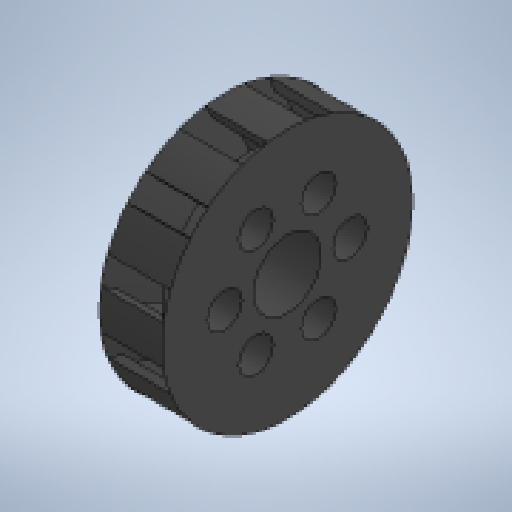
# Autodesk Inventor part: Idler - Hub
Saved by Autodesk Inventor 2023.2 (Build 272271000, 271)
## iProperties
Created: 2023-11-16
Part Number: Idler - Hub
Material: Nylon 6/6
Document SubType Name: Modeling
Designer: Nathan Cai
Density: 1.13 g/cm^3
Appearance: Rubber - Black
Author: Nathan Cai
Autodesk Inventor part; units mm, degrees
ref_plane "YZ Plane" through (0, 0, 0) normal (1, 0, 0) x (0, 1, 0)
ref_plane "XZ Plane" through (0, 0, 0) normal (0, 1, 0) x (-1, 0, 0)
ref_plane "XY Plane" through (0, 0, 0) normal (0, 0, 1) x (1, 0, 0)
sketch "Sketch1" plane through (0, 0, 0) normal (0, 0, 1) x (1, 0, 0)
  line L0 (-3.175, -12.7) -> (3.175, -12.7)
  line L1 (3.175, -12.7) -> (3.175, 12.7)
  line L2 (3.175, 12.7) -> (-3.175, 12.7)
  line L3 (-3.175, 12.7) -> (-3.175, -12.7)
  line L4 (-3.175, -12.7) -> (3.175, 12.7) construction
  line L5 (3.175, -12.7) -> (-3.175, 12.7) construction
  line L6 (-3.175, 0) -> (3.175, 0) construction
  line L7 (-3.175, -3.429) -> (3.175, -3.429)
  line L8 (3.175, -3.429) -> (3.175, 3.429)
  line L9 (3.175, 3.429) -> (-3.175, 3.429)
  line L10 (-3.175, 3.429) -> (-3.175, -3.429)
  line L11 (-3.175, -3.429) -> (3.175, 3.429) construction
  line L12 (3.175, -3.429) -> (-3.175, 3.429) construction
  line L13 (-1.5875, 9.525) -> (1.5875, 9.525)
  line L14 (1.5875, 9.525) -> (1.5875, 15.875)
  line L15 (1.5875, 15.875) -> (-1.5875, 15.875)
  line L16 (-1.5875, 15.875) -> (-1.5875, 9.525)
  line L17 (-1.5875, 9.525) -> (1.5875, 15.875) construction
  line L18 (1.5875, 9.525) -> (-1.5875, 15.875) construction
  point P0 (0, 0)
  point P1 (0, 12.7)
  point P2 (-1.5875, 12.7)
  point P3 (1.5875, 12.7)
  dimension "d0" = 6.35
  dimension "d1" = 25.4
  dimension "d2" = 6.35
  dimension "d3" = 6.858
  dimension "d4" = 3.175
  dimension "d5" = 6.35
  constraints: 38 end point, 9 midpoint, 6 parallel, 3 horizontal, 3 perpendicular
  measures "d0" distance of L2.end L1.end
  measures "d1" distance of L1.end L0.end
  measures "d2" distance of L9.end L8.end
  measures "d3" distance of L8.end L7.end
  measures "d4" distance of L15.end L14.end
  measures "d5" distance of L14.end L13.end
revolve "Revolution1" add sketch "Sketch1" angle 360 about axis through (-3.175, 0, 0) along (1, 0, 0) contours L3 L2 L16 L13 L14 L1 L9
chamfer "Chamfer1" distance 1.5875 angle 45 4 edges at (-1.5875, -12.7, 0) (1.5875, -12.7, 0) (-1.5875, -9.525, 0) (1.5875, -9.525, 0)
sketch "Sketch2" plane through (3.175, 0, 0) normal (1, 0, 0) x (0, 0, -1)
  circle A0 centre (0, 0) radius 9.525
  arc A1 (-11.7597, 1.8625) -> (-11.7597, -1.8625) centre (0, 0) ccw
  circle A2 centre (0, 0) radius 12.7 projected
  line L0 (-12.7, 0) -> (0, 0) construction
  line L1 (-9.5064, -0.5953) -> (-11.8914, -0.5953)
  line L2 (-11.8914, -0.5953) -> (-11.8914, 0.5953) construction
  line L3 (-11.8914, 0.5953) -> (-9.5064, 0.5953)
  line L4 (-9.5064, 0.5953) -> (-9.5064, -0.5953) construction
  line L5 (-9.5064, -0.5953) -> (-11.8914, 0.5953) construction
  line L6 (-11.8914, -0.5953) -> (-9.5064, 0.5953) construction
  line L7 (0, 0) -> (-12.5436, 1.9867) construction
  line L8 (-11.7597, 1.8625) -> (-12.5436, 1.9867)
  line L9 (-11.7597, -1.8625) -> (-12.5436, -1.9867)
  arc A3 (-11.1154, -4.2668) -> (-9.2529, -7.4928) centre (0, 0) ccw
  line L10 (-7.9351, -5.2687) -> (-10.0006, -6.4612)
  line L11 (-10.0006, -6.4612) -> (-10.5959, -5.4301) construction
  line L12 (-10.5959, -5.4301) -> (-8.5304, -4.2376)
  line L13 (-8.5304, -4.2376) -> (-7.9351, -5.2687) construction
  line L14 (-7.9351, -5.2687) -> (-10.5959, -5.4301) construction
  line L15 (-10.0006, -6.4612) -> (-8.5304, -4.2376) construction
  line L16 (-11.1154, -4.2668) -> (-11.8565, -4.5513)
  line L17 (-9.2529, -7.4928) -> (-9.8698, -7.9924)
  arc A4 (-7.4928, -9.2529) -> (-4.2668, -11.1154) centre (0, 0) ccw
  line L18 (-4.2376, -8.5304) -> (-5.4301, -10.5959)
  line L19 (-5.4301, -10.5959) -> (-6.4612, -10.0006) construction
  line L20 (-6.4612, -10.0006) -> (-5.2687, -7.9351)
  line L21 (-5.2687, -7.9351) -> (-4.2376, -8.5304) construction
  line L22 (-4.2376, -8.5304) -> (-6.4612, -10.0006) construction
  line L23 (-5.4301, -10.5959) -> (-5.2687, -7.9351) construction
  line L24 (-7.4928, -9.2529) -> (-7.9924, -9.8698)
  line L25 (-4.2668, -11.1154) -> (-4.5513, -11.8565)
  arc A5 (-1.8625, -11.7597) -> (1.8625, -11.7597) centre (0, 0) ccw
  line L26 (0.5953, -9.5064) -> (0.5953, -11.8914)
  line L27 (0.5953, -11.8914) -> (-0.5953, -11.8914) construction
  line L28 (-0.5953, -11.8914) -> (-0.5953, -9.5064)
  line L29 (-0.5953, -9.5064) -> (0.5953, -9.5064) construction
  line L30 (0.5953, -9.5064) -> (-0.5953, -11.8914) construction
  line L31 (0.5953, -11.8914) -> (-0.5953, -9.5064) construction
  line L32 (-1.8625, -11.7597) -> (-1.9867, -12.5436)
  line L33 (1.8625, -11.7597) -> (1.9867, -12.5436)
  arc A6 (4.2668, -11.1154) -> (7.4928, -9.2529) centre (0, 0) ccw
  line L34 (5.2687, -7.9351) -> (6.4612, -10.0006)
  line L35 (6.4612, -10.0006) -> (5.4301, -10.5959) construction
  line L36 (5.4301, -10.5959) -> (4.2376, -8.5304)
  line L37 (4.2376, -8.5304) -> (5.2687, -7.9351) construction
  line L38 (5.2687, -7.9351) -> (5.4301, -10.5959) construction
  line L39 (6.4612, -10.0006) -> (4.2376, -8.5304) construction
  line L40 (4.2668, -11.1154) -> (4.5513, -11.8565)
  line L41 (7.4928, -9.2529) -> (7.9924, -9.8698)
  arc A7 (9.2529, -7.4928) -> (11.1154, -4.2668) centre (0, 0) ccw
  line L42 (8.5304, -4.2376) -> (10.5959, -5.4301)
  line L43 (10.5959, -5.4301) -> (10.0006, -6.4612) construction
  line L44 (10.0006, -6.4612) -> (7.9351, -5.2687)
  line L45 (7.9351, -5.2687) -> (8.5304, -4.2376) construction
  line L46 (8.5304, -4.2376) -> (10.0006, -6.4612) construction
  line L47 (10.5959, -5.4301) -> (7.9351, -5.2687) construction
  line L48 (9.2529, -7.4928) -> (9.8698, -7.9924)
  line L49 (11.1154, -4.2668) -> (11.8565, -4.5513)
  arc A8 (11.7597, -1.8625) -> (11.7597, 1.8625) centre (0, 0) ccw
  line L50 (9.5064, 0.5953) -> (11.8914, 0.5953)
  line L51 (11.8914, 0.5953) -> (11.8914, -0.5953) construction
  line L52 (11.8914, -0.5953) -> (9.5064, -0.5953)
  line L53 (9.5064, -0.5953) -> (9.5064, 0.5953) construction
  line L54 (9.5064, 0.5953) -> (11.8914, -0.5953) construction
  line L55 (11.8914, 0.5953) -> (9.5064, -0.5953) construction
  line L56 (11.7597, -1.8625) -> (12.5436, -1.9867)
  line L57 (11.7597, 1.8625) -> (12.5436, 1.9867)
  arc A9 (11.1154, 4.2668) -> (9.2529, 7.4928) centre (0, 0) ccw
  line L58 (7.9351, 5.2687) -> (10.0006, 6.4612)
  line L59 (10.0006, 6.4612) -> (10.5959, 5.4301) construction
  line L60 (10.5959, 5.4301) -> (8.5304, 4.2376)
  line L61 (8.5304, 4.2376) -> (7.9351, 5.2687) construction
  line L62 (7.9351, 5.2687) -> (10.5959, 5.4301) construction
  line L63 (10.0006, 6.4612) -> (8.5304, 4.2376) construction
  line L64 (11.1154, 4.2668) -> (11.8565, 4.5513)
  line L65 (9.2529, 7.4928) -> (9.8698, 7.9924)
  arc A10 (7.4928, 9.2529) -> (4.2668, 11.1154) centre (0, 0) ccw
  line L66 (4.2376, 8.5304) -> (5.4301, 10.5959)
  line L67 (5.4301, 10.5959) -> (6.4612, 10.0006) construction
  line L68 (6.4612, 10.0006) -> (5.2687, 7.9351)
  line L69 (5.2687, 7.9351) -> (4.2376, 8.5304) construction
  line L70 (4.2376, 8.5304) -> (6.4612, 10.0006) construction
  line L71 (5.4301, 10.5959) -> (5.2687, 7.9351) construction
  line L72 (7.4928, 9.2529) -> (7.9924, 9.8698)
  line L73 (4.2668, 11.1154) -> (4.5513, 11.8565)
  arc A11 (1.8625, 11.7597) -> (-1.8625, 11.7597) centre (0, 0) ccw
  line L74 (-0.5953, 9.5064) -> (-0.5953, 11.8914)
  line L75 (-0.5953, 11.8914) -> (0.5953, 11.8914) construction
  line L76 (0.5953, 11.8914) -> (0.5953, 9.5064)
  line L77 (0.5953, 9.5064) -> (-0.5953, 9.5064) construction
  line L78 (-0.5953, 9.5064) -> (0.5953, 11.8914) construction
  line L79 (-0.5953, 11.8914) -> (0.5953, 9.5064) construction
  line L80 (1.8625, 11.7597) -> (1.9867, 12.5436)
  line L81 (-1.8625, 11.7597) -> (-1.9867, 12.5436)
  arc A12 (-4.2668, 11.1154) -> (-7.4928, 9.2529) centre (0, 0) ccw
  line L82 (-5.2687, 7.9351) -> (-6.4612, 10.0006)
  line L83 (-6.4612, 10.0006) -> (-5.4301, 10.5959) construction
  line L84 (-5.4301, 10.5959) -> (-4.2376, 8.5304)
  line L85 (-4.2376, 8.5304) -> (-5.2687, 7.9351) construction
  line L86 (-5.2687, 7.9351) -> (-5.4301, 10.5959) construction
  line L87 (-6.4612, 10.0006) -> (-4.2376, 8.5304) construction
  line L88 (-4.2668, 11.1154) -> (-4.5513, 11.8565)
  line L89 (-7.4928, 9.2529) -> (-7.9924, 9.8698)
  arc A13 (-9.2529, 7.4928) -> (-11.1154, 4.2668) centre (0, 0) ccw
  line L90 (-8.5304, 4.2376) -> (-10.5959, 5.4301)
  line L91 (-10.5959, 5.4301) -> (-10.0006, 6.4612) construction
  line L92 (-10.0006, 6.4612) -> (-7.9351, 5.2687)
  line L93 (-7.9351, 5.2687) -> (-8.5304, 4.2376) construction
  line L94 (-8.5304, 4.2376) -> (-10.0006, 6.4612) construction
  line L95 (-10.5959, 5.4301) -> (-7.9351, 5.2687) construction
  line L96 (-9.2529, 7.4928) -> (-9.8698, 7.9924)
  line L97 (-11.1154, 4.2668) -> (-11.8565, 4.5513)
  circle A14 centre (0, 0) radius 3.429
  point P0 (-10.6989, 0)
  point P1 (-10.9985, -6.35)
  point P2 (-9.2655, -5.3494)
  point P3 (-6.35, -10.9985)
  point P4 (-5.3494, -9.2655)
  point P5 (0, -12.7)
  point P6 (0, -10.6989)
  point P7 (6.35, -10.9985)
  point P8 (5.3494, -9.2655)
  point P9 (10.9985, -6.35)
  point P10 (9.2655, -5.3494)
  point P11 (12.7, 0)
  point P12 (10.6989, 0)
  point P13 (10.9985, 6.35)
  point P14 (9.2655, 5.3494)
  point P15 (6.35, 10.9985)
  point P16 (5.3494, 9.2655)
  point P17 (0, 12.7)
  point P18 (0, 10.6989)
  point P19 (-6.35, 10.9985)
  point P20 (-5.3494, 9.2655)
  point P21 (-10.9985, 6.35)
  point P22 (-9.2655, 5.3494)
  dimension "d10" = 19.05
  dimension "d11" = 0.7937
  dimension "d12" = 1.1906
  dimension "d13" = 9
  dimension "d16" = 360
  dimension "d20" = 6.858
  constraints: 196 end point, 36 point on circle, 13 centre point, 3 coincident, 2 horizontal, 2 midpoint, 2 parallel, 2 point on line, 2 symmetric about line, 1 collinear, 1 perpendicular, 247 other
  measures "d12" distance between parallel lines of L1 L3
  measures "d13" angle of L0 L7
  measures "d20" diameter of A14
extrude "Extrusion1" add sketch "Sketch2" against normal up to surface (6.35 mm away) contours A0 | A0 L50 A8 L52 | A0 L58 A9 L60 | A8 L57 A2 L56 | L42 A7 L44 A0 | A9 L65 A2 L64 | A7 L49 A2 L48 | A0 L66 A10 L68 | L34 A6 L36 A0 | A10 L73 A2 L72 | A6 L41 A2 L40 | A0 L74 A11 L76 | L26 A5 L28 A0 | A11 L81 A2 L80 | A5 L33 A2 L32 | A0 L82 A12 L84 | L18 A4 L20 A0 | A12 L89 A2 L88 | A4 L25 A2 L24 | A0 L90 A13 L92 | L10 A3 L12 A0 | A13 L97 A2 L96 | A3 L17 A2 L16 | A0 L1 A1 L3 | A1 L9 A2 L8
sketch "Sketch3" plane through (3.175, 0, 0) normal (1, 0, 0) x (0, 0, -1)
  arc A0 (-7.9924, -9.8698) -> (-4.5513, -11.8565) centre (0, 0) ccw projected
  circle A1 centre (0, 0) radius 6.35 construction
  line L0 (-6.35, 0) -> (0, 0) construction
  circle A2 centre (-6.35, 0) radius 1.7526
  circle A3 centre (-3.175, -5.4993) radius 1.7526
  circle A4 centre (3.175, -5.4993) radius 1.7526
  circle A5 centre (6.35, 0) radius 1.7526
  circle A6 centre (3.175, 5.4993) radius 1.7526
  circle A7 centre (-3.175, 5.4993) radius 1.7526
  dimension "d21" = 12.7
  dimension "d22" = 3.5052
  dimension "d25" = 360
  constraints: 6 centre point, 2 coincident, 2 end point, 1 horizontal, 1 horizontal alignment, 15 other
  measures "d22" diameter of A2
extrude "Extrusion2" cut sketch "Sketch3" against normal through all
body "Solid1"
